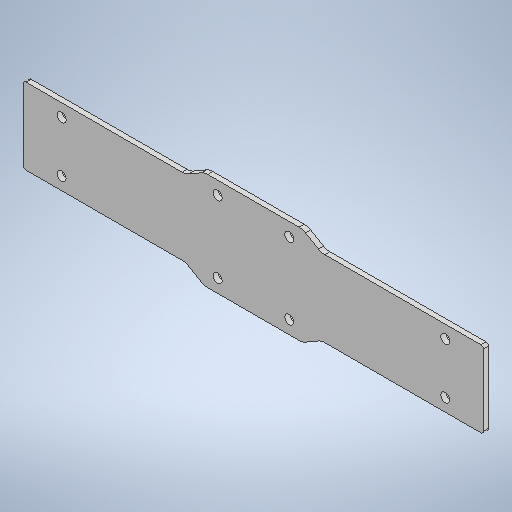
# Autodesk Inventor part: T2.0_frame-base4
Saved by Autodesk Inventor 2025 (Build 290162000, 162)
## iProperties
Created: 2024-06-30
Part Number: T2.0_frame-base4
Material: 一般
Document SubType Name: Sheet Metal
Designer: 8326d
Density: 1 g/cm^3
Sheet Metal Rule: Default_mm
Appearance: 既定
Author: 8326d
Autodesk Inventor part; units mm, degrees
ref_plane "YZ Plane" through (0, 0, 0) normal (1, 0, 0) x (0, 1, 0)
ref_plane "XZ Plane" through (0, 0, 0) normal (0, 1, 0) x (-1, 0, 0)
ref_plane "XY Plane" through (0, 0, 0) normal (0, 0, 1) x (1, 0, 0)
sketch "スケッチ1" plane through (0, 0, 0) normal (0, 0, 1) x (1, 0, 0)
  line L0 (-90.5, -15) -> (90.5, -15)
  line L1 (90.5, -15) -> (90.5, 15)
  line L2 (90.5, 15) -> (-90.5, 15)
  line L3 (-90.5, 15) -> (-90.5, -15)
  line L4 (-90.5, -15) -> (90.5, 15) construction
  line L5 (90.5, -15) -> (-90.5, 15) construction
  line L6 (-19.3, -19.3) -> (19.3, -19.3)
  line L7 (19.3, -19.3) -> (19.3, 19.3)
  line L8 (19.3, 19.3) -> (-19.3, 19.3)
  line L9 (-19.3, 19.3) -> (-19.3, -19.3)
  line L10 (-19.3, -19.3) -> (19.3, 19.3) construction
  line L11 (19.3, -19.3) -> (-19.3, 19.3) construction
  line L12 (-19.3, 19.3) -> (-26.7478, 15)
  line L13 (-19.3, -19.3) -> (-26.7478, -15)
  line L14 (19.3, -19.3) -> (26.7478, -15)
  line L15 (26.7478, 15) -> (19.3, 19.3)
  point P0 (0, 0)
  dimension "d0" = 181
  dimension "d1" = 30
  dimension "d2" = 38.6
  dimension "d3" = 38.6
  dimension "d4" = 150
  dimension "d5" = 150
  measures "d0" distance of L2.end L1.end
  measures "d1" distance of L1.end L0.end
  measures "d2" distance of L8.end L7.end
  measures "d3" distance of L7.end L6.end
  measures "d4" angle of L2 L15
  measures "d5" angle of L0 L14
extrude "プレート1" add sketch "スケッチ1" along normal blind 2
sketch "スケッチ2" plane through (0, 0, 2) normal (0, 0, 1) x (1, 0, 0)
  line L0 (-75.5, -10) -> (75.5, -10) construction
  line L1 (75.5, -10) -> (75.5, 10) construction
  line L2 (75.5, 10) -> (-75.5, 10) construction
  line L3 (-75.5, 10) -> (-75.5, -10) construction
  line L4 (-75.5, -10) -> (75.5, 10) construction
  line L5 (75.5, -10) -> (-75.5, 10) construction
  point P0 (0, 0)
  dimension "d7" = 151
  dimension "d8" = 20
  constraints: 12 end point, 2 midpoint, 2 parallel, 1 horizontal, 1 perpendicular
  measures "d7" distance of L2.end L1.end
  measures "d8" distance of L1.end L0.end
hole "穴1" at (-75.5, 10, 2) at (-75.5, -10, 2) at (75.5, -10, 2) at (75.5, 10, 2) direction (0, 0, -1) diameter 3.5 depth 2 tip angle 118
sketch "スケッチ3" plane through (0, 0, 2) normal (0, 0, 1) x (1, 0, 0)
  line L0 (-14.1, -14.1) -> (14.1, -14.1) construction
  line L1 (14.1, -14.1) -> (14.1, 14.1) construction
  line L2 (14.1, 14.1) -> (-14.1, 14.1) construction
  line L3 (-14.1, 14.1) -> (-14.1, -14.1) construction
  line L4 (-14.1, -14.1) -> (14.1, 14.1) construction
  line L5 (14.1, -14.1) -> (-14.1, 14.1) construction
  point P0 (0, 0)
  dimension "d16" = 28.2
  dimension "d17" = 28.2
  constraints: 12 end point, 2 midpoint, 2 parallel, 1 horizontal, 1 perpendicular
  measures "d16" distance of L2.end L1.end
  measures "d17" distance of L1.end L0.end
hole "穴2" at (14.1, 14.1, 2) at (14.1, -14.1, 2) at (-14.1, -14.1, 2) at (-14.1, 14.1, 2) direction (0, 0, -1) diameter 3.5 depth 2 tip angle 118
fillet "フィレット1" radius 5 8 edges at (26.7478, 15, 1) (19.3, 19.3, 1) (26.7478, -15, 1) (19.3, -19.3, 1) (-19.3, -19.3, 1) (-26.7478, -15, 1) (-26.7478, 15, 1) (-19.3, 19.3, 1)
fillet "フィレット2" radius 1 4 edges at (-90.5, 15, 1) (-90.5, -15, 1) (90.5, -15, 1) (90.5, 15, 1)
equation "\"d3\" = d2"
equation "\"d5\" = d4"
equation "\"d14\" = Thickness"
equation "\"d23\" = Thickness"
equation "\"d6\" = Thickness"
equation "\"BendRadius\" = Thickness"
equation "\"BendReliefWidth\" = Thickness"
equation "\"BendReliefDepth\" = 0.5 * Thickness"
equation "\"CornerReliefSize\" = 4 * Thickness"
equation "\"MinimumRemnant\" = 2 * Thickness"
equation "\"TransitionRadius\" = BendRadius"
equation "\"JacobiRadiusSize\" = BendRadius"
equation "\"GapSize\" = Thickness"
equation "\"Thickness\" = 2"
